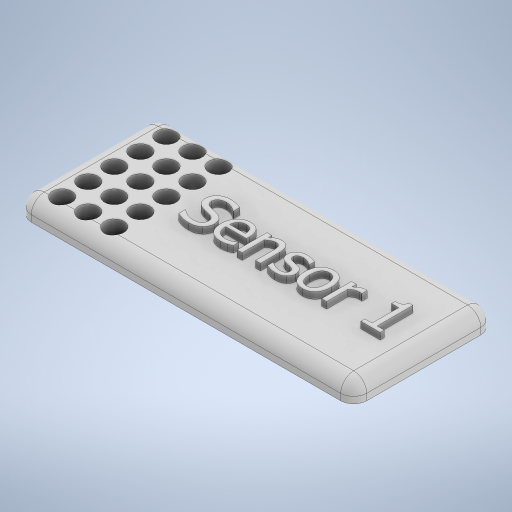
# Autodesk Inventor part: sensor1
Saved by Autodesk Inventor 2024 (Build 280153000, 153)
## iProperties
Created: 2024-03-06
Part Number: sensor1
Material: Generic
Document SubType Name: Modeling
Designer: quinten
Density: 1 g/cm^3
Appearance: Default
Author: quinten
Autodesk Inventor part; units mm, degrees
ref_plane "YZ Plane" through (0, 0, 0) normal (1, 0, 0) x (0, 1, 0)
ref_plane "XZ Plane" through (0, 0, 0) normal (0, 1, 0) x (-1, 0, 0)
ref_plane "XY Plane" through (0, 0, 0) normal (0, 0, 1) x (1, 0, 0)
sketch "Sketch1" plane through (0, 0, 0) normal (0, 1, 0) x (-1, 0, 0)
  line L0 (0, 0) -> (51.5, 0)
  line L1 (51.5, 0) -> (51.5, -21.5)
  line L2 (51.5, -21.5) -> (0, -21.5)
  line L3 (0, -21.5) -> (0, 0)
  line L4 (51.5, -10.75) -> (0, -10.75) construction
  line L5 (47.5, 0) -> (47.5, -21.5) construction
  circle A0 centre (47.5, -2.75) radius 1.5
  circle A1 centre (47.5, -10.75) radius 1.5
  circle A2 centre (47.5, -6.75) radius 1.5
  circle A3 centre (47.5, -14.75) radius 1.5
  circle A4 centre (47.5, -18.75) radius 1.5
  circle A5 centre (43.5, -2.75) radius 1.5
  circle A6 centre (43.5, -6.75) radius 1.5
  circle A7 centre (43.5, -10.75) radius 1.5
  circle A8 centre (43.5, -14.75) radius 1.5
  circle A9 centre (43.5, -18.75) radius 1.5
  circle A10 centre (39.5, -2.75) radius 1.5
  circle A11 centre (39.5, -6.75) radius 1.5
  circle A12 centre (39.5, -10.75) radius 1.5
  circle A13 centre (39.5, -14.75) radius 1.5
  circle A14 centre (39.5, -18.75) radius 1.5
  dimension "d0" = 51.5
  dimension "d1" = 21.5
  dimension "d2" = 4
  dimension "d3" = 3
  dimension "d4" = 3
  dimension "d5" = 3
  dimension "d6" = 3
  dimension "d7" = 3
  dimension "d8" = 4
  dimension "d9" = 4
  dimension "d10" = 4
  dimension "d11" = 4
  dimension "d14" = 4
  constraints: 15 centre point, 12 end point, 6 point on line, 3 midpoint, 2 horizontal, 2 parallel, 2 perpendicular, 20 other
  measures "d0" distance of L1.end L2.end
  measures "d1" distance of L0.end L1.end
  measures "d2" distance between parallel lines of L1 L5
  measures "d3" diameter of A0
  measures "d4" diameter of A1
  measures "d5" diameter of A2
  measures "d6" diameter of A3
  measures "d7" diameter of A4
  measures "d8" distance of A1.centre A3.centre
  measures "d9" distance of A3.centre A4.centre
  measures "d10" distance of A1.centre A2.centre
  measures "d11" distance of A2.centre A0.centre
  measures "d14" distance of A0.centre A5.centre
extrude "Extrusion1" add sketch "Sketch1" along normal blind 3
fillet "Fillet1" radius 2 8 edges at (0, 1.5, 0) (-25.75, 3, 0) (0, 3, -10.75) (0, 1.5, -21.5) (-25.75, 3, -21.5) (-51.5, 3, -10.75) (-51.5, 1.5, 0) (-51.5, 1.5, -21.5)
sketch "Sketch2" plane through (0, 3, 0) normal (0, 1, 0) x (1, 0, 0)
  line L0 (-35.6591, 14.3268) -> (-1.7873, 14.3268) construction
  line L1 (-1.7873, 14.3268) -> (-1.7873, 6.1649) construction
  line L2 (-1.7873, 6.1649) -> (-35.6591, 6.1649) construction
  line L3 (-35.6591, 6.1649) -> (-35.6591, 14.3268) construction
  spline S0 degree 2 poles (-33.3407, 8.0092) (-34.0031, 8.0092) (-34.9325, 8.2861) (-35.3428, 8.4838) knots 0 0 0 1 2 2 2
  line L4 (-35.3428, 8.4838) -> (-35.3428, 9.5021)
  line L5 (-35.3428, 9.5021) -> (-35.2834, 9.5021)
  spline S1 degree 2 poles (-35.2834, 9.5021) (-34.883, 9.1264) (-33.8697, 8.7112) (-33.4, 8.7112) knots 0 0 0 1 2 2 2
  spline S2 degree 2 poles (-33.4, 8.7112) (-32.7278, 8.7112) (-32.0406, 9.2698) (-32.0406, 9.7295) knots 0 0 0 1 2 2 2
  spline S3 degree 2 poles (-32.0406, 9.7295) (-32.0406, 10.0953) (-32.4015, 10.5501) (-32.792, 10.6638) knots 0 0 0 1 2 2 2
  spline S4 degree 2 poles (-32.792, 10.6638) (-33.0738, 10.7429) (-33.5434, 10.8516) (-33.8944, 10.9406) knots 0 0 0 1 2 2 2
  spline S5 degree 2 poles (-33.8944, 10.9406) (-34.2107, 11.0246) (-34.71, 11.2768) (-34.9028, 11.4794) knots 0 0 0 1 2 2 2
  spline S6 degree 2 poles (-34.9028, 11.4794) (-35.0906, 11.6821) (-35.2983, 12.2259) (-35.2983, 12.5818) knots 0 0 0 1 2 2 2
  spline S7 degree 2 poles (-35.2983, 12.5818) (-35.2983, 13.3233) (-34.1415, 14.3268) (-33.2468, 14.3268) knots 0 0 0 1 2 2 2
  spline S8 degree 2 poles (-33.2468, 14.3268) (-32.7327, 14.3268) (-31.8231, 14.1241) (-31.4326, 13.9313) knots 0 0 0 1 2 2 2
  line L6 (-31.4326, 13.9313) -> (-31.4326, 12.9624)
  line L7 (-31.4326, 12.9624) -> (-31.4919, 12.9624)
  spline S9 degree 2 poles (-31.4919, 12.9624) (-31.7836, 13.2293) (-32.6932, 13.6248) (-33.1924, 13.6248) knots 0 0 0 1 2 2 2
  spline S10 degree 2 poles (-33.1924, 13.6248) (-33.756, 13.6248) (-34.453, 13.0959) (-34.453, 12.6658) knots 0 0 0 1 2 2 2
  spline S11 degree 2 poles (-34.453, 12.6658) (-34.453, 12.2802) (-34.0427, 11.8205) (-33.6571, 11.7167) knots 0 0 0 1 2 2 2
  spline S12 degree 2 poles (-33.6571, 11.7167) (-33.4, 11.6475) (-32.6536, 11.4695) (-32.4064, 11.3954) knots 0 0 0 1 2 2 2
  spline S13 degree 2 poles (-32.4064, 11.3954) (-31.7787, 11.2026) (-31.1953, 10.4265) (-31.1953, 9.858) knots 0 0 0 1 2 2 2
  spline S14 degree 2 poles (-31.1953, 9.858) (-31.1953, 9.4972) (-31.487, 8.8051) (-31.749, 8.5629) knots 0 0 0 1 2 2 2
  spline S15 degree 2 poles (-31.749, 8.5629) (-32.0406, 8.296) (-32.7821, 8.0092) (-33.3407, 8.0092) knots 0 0 0 1 2 2 2
  spline S16 degree 2 poles (-28.4419, 8.0142) (-29.5393, 8.0142) (-30.7455, 9.2451) (-30.7455, 10.382) knots 0 0 0 1 2 2 2
  spline S17 degree 2 poles (-30.7455, 10.382) (-30.7455, 11.4992) (-29.574, 12.824) (-28.6298, 12.824) knots 0 0 0 1 2 2 2
  spline S18 degree 2 poles (-28.6298, 12.824) (-28.2047, 12.824) (-27.5472, 12.5768) (-27.305, 12.3148) knots 0 0 0 1 2 2 2
  spline S19 degree 2 poles (-27.305, 12.3148) (-27.0578, 12.0528) (-26.7958, 11.2965) (-26.7958, 10.7478) knots 0 0 0 1 2 2 2
  line L8 (-26.7958, 10.7478) -> (-26.7958, 10.3276)
  line L9 (-26.7958, 10.3276) -> (-29.9645, 10.3276)
  spline S20 degree 2 poles (-29.9645, 10.3276) (-29.9645, 9.5318) (-29.1637, 8.6865) (-28.4518, 8.6865) knots 0 0 0 1 2 2 2
  spline S21 degree 2 poles (-28.4518, 8.6865) (-28.1997, 8.6865) (-27.7103, 8.8002) (-27.5126, 8.8892) knots 0 0 0 1 2 2 2
  spline S22 degree 2 poles (-27.5126, 8.8892) (-27.305, 8.988) (-27.0183, 9.161) (-26.9244, 9.2401) knots 0 0 0 1 2 2 2
  line L10 (-26.9244, 9.2401) -> (-26.8799, 9.2401)
  line L11 (-26.8799, 9.2401) -> (-26.8799, 8.3998)
  spline S23 degree 2 poles (-26.8799, 8.3998) (-27.0133, 8.3454) (-27.4187, 8.1872) (-27.5769, 8.1427) knots 0 0 0 1 2 2 2
  spline S24 degree 2 poles (-27.5769, 8.1427) (-27.7993, 8.0785) (-28.1651, 8.0142) (-28.4419, 8.0142) knots 0 0 0 1 2 2 2
  spline S25 degree 2 poles (-27.5472, 10.9159) (-27.5571, 11.2273) (-27.6856, 11.6821) (-27.8092, 11.8353) knots 0 0 0 1 2 2 2
  spline S26 degree 2 poles (-27.8092, 11.8353) (-27.9427, 12.0084) (-28.3628, 12.1913) (-28.6743, 12.1913) knots 0 0 0 1 2 2 2
  spline S27 degree 2 poles (-28.6743, 12.1913) (-28.9808, 12.1913) (-29.4108, 12.0084) (-29.5888, 11.8304) knots 0 0 0 1 2 2 2
  spline S28 degree 2 poles (-29.5888, 11.8304) (-29.7618, 11.6475) (-29.9398, 11.2075) (-29.9645, 10.9159) knots 0 0 0 1 2 2 2
  line L12 (-29.9645, 10.9159) -> (-27.5472, 10.9159)
  line L13 (-22.421, 8.118) -> (-23.1922, 8.118)
  line L14 (-23.1922, 8.118) -> (-23.1922, 10.728)
  spline S29 degree 2 poles (-23.1922, 10.728) (-23.1922, 11.0444) (-23.2515, 11.5882) (-23.3405, 11.7513) knots 0 0 0 1 2 2 2
  spline S30 degree 2 poles (-23.3405, 11.7513) (-23.4344, 11.9243) (-23.7705, 12.0924) (-24.0573, 12.0924) knots 0 0 0 1 2 2 2
  spline S31 degree 2 poles (-24.0573, 12.0924) (-24.344, 12.0924) (-24.952, 11.7859) (-25.2436, 11.5387) knots 0 0 0 1 2 2 2
  line L15 (-25.2436, 11.5387) -> (-25.2436, 8.118)
  line L16 (-25.2436, 8.118) -> (-26.0148, 8.118)
  line L17 (-26.0148, 8.118) -> (-26.0148, 12.6955)
  line L18 (-26.0148, 12.6955) -> (-25.2436, 12.6955)
  line L19 (-25.2436, 12.6955) -> (-25.2436, 12.1863)
  spline S32 degree 2 poles (-25.2436, 12.1863) (-24.8976, 12.4977) (-24.2303, 12.824) (-23.8546, 12.824) knots 0 0 0 1 2 2 2
  spline S33 degree 2 poles (-23.8546, 12.824) (-23.1823, 12.824) (-22.421, 11.9342) (-22.421, 11.0889) knots 0 0 0 1 2 2 2
  line L20 (-22.421, 11.0889) -> (-22.421, 8.118)
  spline S34 degree 2 poles (-20.1026, 8.0092) (-20.5624, 8.0092) (-21.3582, 8.2564) (-21.6202, 8.3948) knots 0 0 0 1 2 2 2
  line L21 (-21.6202, 8.3948) -> (-21.6202, 9.2599)
  line L22 (-21.6202, 9.2599) -> (-21.5807, 9.2599)
  spline S35 degree 2 poles (-21.5807, 9.2599) (-21.4818, 9.1808) (-21.2149, 8.993) (-20.9924, 8.8892) knots 0 0 0 1 2 2 2
  spline S36 degree 2 poles (-20.9924, 8.8892) (-20.7996, 8.7952) (-20.3251, 8.6568) (-20.073, 8.6568) knots 0 0 0 1 2 2 2
  spline S37 degree 2 poles (-20.073, 8.6568) (-19.8901, 8.6568) (-19.4699, 8.7409) (-19.371, 8.8101) knots 0 0 0 1 2 2 2
  spline S38 degree 2 poles (-19.371, 8.8101) (-19.2277, 8.904) (-19.0992, 9.1165) (-19.0992, 9.334) knots 0 0 0 1 2 2 2
  spline S39 degree 2 poles (-19.0992, 9.334) (-19.0992, 9.6059) (-19.3957, 9.8877) (-19.7764, 9.9816) knots 0 0 0 1 2 2 2
  spline S40 degree 2 poles (-19.7764, 9.9816) (-19.9247, 10.0162) (-20.3992, 10.1151) (-20.6019, 10.1695) knots 0 0 0 1 2 2 2
  spline S41 degree 2 poles (-20.6019, 10.1695) (-21.1259, 10.3227) (-21.6005, 10.9554) (-21.6005, 11.4053) knots 0 0 0 1 2 2 2
  spline S42 degree 2 poles (-21.6005, 11.4053) (-21.6005, 12.0281) (-20.6662, 12.8042) (-19.895, 12.8042) knots 0 0 0 1 2 2 2
  spline S43 degree 2 poles (-19.895, 12.8042) (-19.5144, 12.8042) (-18.7432, 12.6164) (-18.4812, 12.473) knots 0 0 0 1 2 2 2
  line L23 (-18.4812, 12.473) -> (-18.4812, 11.6475)
  line L24 (-18.4812, 11.6475) -> (-18.5208, 11.6475)
  spline S44 degree 2 poles (-18.5208, 11.6475) (-18.8174, 11.8848) (-19.5391, 12.1567) (-19.9099, 12.1567) knots 0 0 0 1 2 2 2
  spline S45 degree 2 poles (-19.9099, 12.1567) (-20.2905, 12.1567) (-20.8145, 11.8353) (-20.8145, 11.514) knots 0 0 0 1 2 2 2
  spline S46 degree 2 poles (-20.8145, 11.514) (-20.8145, 11.2224) (-20.503, 10.9406) (-20.157, 10.8516) knots 0 0 0 1 2 2 2
  spline S47 degree 2 poles (-20.157, 10.8516) (-19.9889, 10.8071) (-19.5638, 10.7182) (-19.3315, 10.6638) knots 0 0 0 1 2 2 2
  spline S48 degree 2 poles (-19.3315, 10.6638) (-18.8273, 10.5353) (-18.3132, 9.947) (-18.3132, 9.4379) knots 0 0 0 1 2 2 2
  spline S49 degree 2 poles (-18.3132, 9.4379) (-18.3132, 9.1413) (-18.5455, 8.6173) (-18.7729, 8.4245) knots 0 0 0 1 2 2 2
  spline S50 degree 2 poles (-18.7729, 8.4245) (-19.0151, 8.2218) (-19.633, 8.0092) (-20.1026, 8.0092) knots 0 0 0 1 2 2 2
  spline S51 degree 2 poles (-13.8346, 10.4067) (-13.8346, 9.25) (-14.9468, 7.9895) (-15.8761, 7.9895) knots 0 0 0 1 2 2 2
  spline S52 degree 2 poles (-15.8761, 7.9895) (-16.8302, 7.9895) (-17.9227, 9.2896) (-17.9227, 10.4067) knots 0 0 0 1 2 2 2
  spline S53 degree 2 poles (-17.9227, 10.4067) (-17.9227, 11.5536) (-16.7956, 12.824) (-15.8761, 12.824) knots 0 0 0 1 2 2 2
  spline S54 degree 2 poles (-15.8761, 12.824) (-14.9468, 12.824) (-13.8346, 11.5585) (-13.8346, 10.4067) knots 0 0 0 1 2 2 2
  spline S55 degree 2 poles (-14.6304, 10.4067) (-14.6304, 11.2965) (-15.278, 12.1616) (-15.8761, 12.1616) knots 0 0 0 1 2 2 2
  spline S56 degree 2 poles (-15.8761, 12.1616) (-16.4743, 12.1616) (-17.1268, 11.2965) (-17.1268, 10.4067) knots 0 0 0 1 2 2 2
  spline S57 degree 2 poles (-17.1268, 10.4067) (-17.1268, 9.5417) (-16.4743, 8.6519) (-15.8761, 8.6519) knots 0 0 0 1 2 2 2
  spline S58 degree 2 poles (-15.8761, 8.6519) (-15.2829, 8.6519) (-14.6304, 9.5268) (-14.6304, 10.4067) knots 0 0 0 1 2 2 2
  line L25 (-10.6165, 11.8699) -> (-10.656, 11.8699)
  spline S59 degree 2 poles (-10.656, 11.8699) (-10.745, 11.8947) (-10.9378, 11.9045) (-11.0713, 11.9045) knots 0 0 0 1 2 2 2
  spline S60 degree 2 poles (-11.0713, 11.9045) (-11.3827, 11.9045) (-11.9957, 11.6327) (-12.2725, 11.3657) knots 0 0 0 1 2 2 2
  line L26 (-12.2725, 11.3657) -> (-12.2725, 8.118)
  line L27 (-12.2725, 8.118) -> (-13.0436, 8.118)
  line L28 (-13.0436, 8.118) -> (-13.0436, 12.6955)
  line L29 (-13.0436, 12.6955) -> (-12.2725, 12.6955)
  line L30 (-12.2725, 12.6955) -> (-12.2725, 12.0133)
  spline S61 degree 2 poles (-12.2725, 12.0133) (-11.8523, 12.389) (-11.2245, 12.6955) (-10.9279, 12.6955) knots 0 0 0 1 2 2 2
  spline S62 degree 2 poles (-10.9279, 12.6955) (-10.8093, 12.6955) (-10.6906, 12.6856) (-10.6165, 12.6708) knots 0 0 0 1 2 2 2
  line L31 (-10.6165, 12.6708) -> (-10.6165, 11.8699)
  line L32 (-4.0568, 8.118) -> (-7.0326, 8.118)
  line L33 (-7.0326, 8.118) -> (-7.0326, 8.7409)
  line L34 (-7.0326, 8.7409) -> (-5.9253, 8.7409)
  line L35 (-5.9253, 8.7409) -> (-5.9253, 12.8289)
  line L36 (-5.9253, 12.8289) -> (-7.0326, 12.8289)
  line L37 (-7.0326, 12.8289) -> (-7.0326, 13.3875)
  spline S63 degree 2 poles (-7.0326, 13.3875) (-6.4048, 13.3875) (-5.8116, 13.7434) (-5.7721, 14.2378) knots 0 0 0 1 2 2 2
  line L38 (-5.7721, 14.2378) -> (-5.1393, 14.2378)
  line L39 (-5.1393, 14.2378) -> (-5.1393, 8.7409)
  line L40 (-5.1393, 8.7409) -> (-4.0568, 8.7409)
  line L41 (-4.0568, 8.7409) -> (-4.0568, 8.118)
  point P0 (0, 0)
  constraints: 2 other
extrude "Extrusion2" add sketch "Sketch2" along normal blind 1
equation "\"d2\" = d9"
equation "\"d3\" = d7"
equation "\"d4\" = d7"
equation "\"d5\" = d7"
equation "\"d6\" = d7"
equation "\"d9\" = d8"
equation "\"d10\" = d9"
equation "\"d11\" = d10"
body "Solid1"
